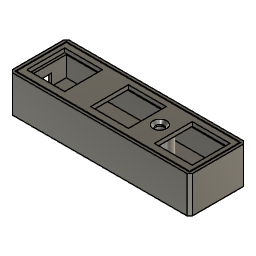
cad (Autodesk Fusion 360 design; units mm, degrees)
Autodesk Fusion 360 part; units mm, degrees
sketch "Sketch1" plane through (0, 0, 0) normal (0, 0, 1) x (1, 0, 0)
  line L0 (0, 0) -> (13.9, 0)
  line L1 (13.9, 0) -> (13.9, 13.9)
  line L2 (13.9, 13.9) -> (0, 13.9)
  line L3 (0, 13.9) -> (0, 0)
  line L4 (0, 6.95) -> (38, 6.95)
  circle A0 centre (42, 6.95) radius 4
  circle A1 centre (42, 6.95) radius 2.5
  line L5 (37.4, 13.9) -> (23.5, 13.9)
  line L6 (37.4, 0) -> (37.4, 13.9)
  line L7 (23.5, 13.9) -> (23.5, 0)
  line L8 (23.5, 0) -> (37.4, 0)
  line L9 (60.9, 13.9) -> (47, 13.9)
  line L10 (60.9, 0) -> (60.9, 13.9)
  line L11 (47, 13.9) -> (47, 0)
  line L12 (47, 0) -> (60.9, 0)
  line L13 (0, 0) -> (0, -0.3232)
  line L14 (0, -0.3232) -> (0, -2.4232)
  line L15 (0, -2.4232) -> (-1.5, -2.4232)
  line L16 (60.9, 13.9) -> (60.9, 16)
  line L17 (60.9, 16) -> (62.4, 16)
  line L18 (62.4, 16) -> (-1.5, 16)
  line L19 (-1.5, 16) -> (-1.5, -2.4232)
  line L20 (-1.5, -2.4232) -> (62.4, -2.4232)
  line L21 (62.4, -2.4232) -> (62.4, 16)
  line L22 (-1.7, -2.6232) -> (62.6, -2.6232)
  line L23 (62.6, -2.6232) -> (62.6, 16.2)
  line L24 (62.6, 16.2) -> (-1.7, 16.2)
  line L25 (-1.7, 16.2) -> (-1.7, -2.6232)
  line L26 (63.6, 17.2) -> (-2.7, 17.2)
  line L27 (-2.7, 17.2) -> (-2.7, -3.6232)
  line L28 (-2.7, -3.6232) -> (63.6, -3.6232)
  line L29 (63.6, -3.6232) -> (63.6, 17.2)
  line L30 (-1.7, -2.6232) -> (-1.7, 5.5768)
  line L31 (-1.7, 5.5768) -> (-1.7, 13.3768)
  circle A2 centre (42, 6.95) radius 1.5
  line L32 (-2.7, 6.7884) -> (-2.7, 2.7884)
  line L33 (-2.7, 2.7884) -> (-1.7, 2.7884)
  line L34 (-1.7, 2.7884) -> (-1.7, 10.7884)
  line L35 (-1.7, 10.7884) -> (-2.7, 10.7884)
  line L36 (-2.7, 10.7884) -> (-2.7, 2.7884)
  line L37 (32.5, 6.7884) -> (32.5, 16.2)
  line L38 (32.5, 16.2) -> (34.5, 16.2)
  line L39 (34.5, 16.2) -> (34.5, -2.3232)
  line L40 (34.5, -2.3232) -> (32.5, -2.3232)
  line L41 (32.5, -2.3232) -> (32.5, 16.2)
  dimension "d1" = 13.9
  dimension "d2" = 13.9
  dimension "d3" = 38
  dimension "d4" = 8
  dimension "d5" = 5
  dimension "d8" = 23.5
  dimension "d9" = 0
  dimension "d10" = 2.1
  dimension "d11" = 1.5
  dimension "d12" = 2.1
  dimension "d13" = 1.5
  dimension "d14" = 0.2
  dimension "d15" = 1.2
  dimension "d18" = 3
  dimension "d47" = 4
  dimension "d48" = 8
  dimension "d58" = 2
  constraint horizontal L0
  constraint vertical L1
  constraint horizontal L2
  constraint vertical L3
  constraint coincident L0.start L3.end
  constraint midpoint L3 L4.start
  constraint perpendicular L1 L4
  constraint coincident L4.end A0
  constraint concentric A0 A1
  constraint perpendicular L0 L13
  constraint perpendicular L0 L14
  constraint perpendicular L14 L15
  constraint perpendicular L9 L16
  constraint perpendicular L16 L17
  constraint horizontal L18
  constraint vertical L19
  constraint horizontal L20
  constraint vertical L21
  constraint perpendicular L22 L30
  constraint parallel L25 L31
  constraint concentric A0 A2
  constraint midpoint L27 L32.start
  constraint perpendicular L28 L32
  constraint horizontal L33
  constraint vertical L34
  constraint horizontal L35
  constraint vertical L36
  constraint coincident L24 L37.end
  constraint perpendicular L18 L37
  constraint horizontal L38
  constraint vertical L39
  constraint horizontal L40
  constraint vertical L41
  measures "d1" distance of L0.start L0.end
  measures "d2" distance of L0.start L2.end
  measures "d3" distance of L4.start L4.end
  measures "d4" diameter of A0
  measures "d5" diameter of A1
  measures "d10" distance of L13.end L14.end
  measures "d11" distance of L14.end L15.end
  measures "d12" distance of L9.start L16.end
  measures "d13" distance of L16.end L17.end
  measures "d18" diameter of A2
  measures "d47" distance of L32.start L32.end
  measures "d48" distance of L32.end L35.end
  measures "d58" distance of L37.end L38.end
extrude "Extrude1" add sketch "Sketch1" along normal blind 1.5 contours L1 L2 L3 L4 L5 L7 L13 L14 L15 L18 L19 L20 L37 L41 | L0 L1 L4 L5 L6 L7 L8 L13 L14 L17 L18 L20 L21 L39 L40 L41 | L5 L18 L37 L39 L41 | L8 L39 L40 L41 | A0 | A1 makes body 1
extrude "Extrude2" add sketch "Sketch1" along normal blind 1.5 and the other way blind 20 separate body contours L22 L23 L24 L25 L26 L27 L28 L29 L30 L31 L33 L35 L38 | L25 L27 L30 L31 L32 L33 L34 L35 L36 makes body 2
extrude "Extrude3" add sketch "Sketch1" along normal blind -22 and the other way blind 20 contours L0 L1 L3 L4 | L1 L2 L3 L4 L5 L7 L13 L14 L15 L18 L19 L20 L37 L41 | L0 L1 L4 L5 L6 L7 L8 L13 L14 L17 L18 L20 L21 L39 L40 L41 | L1 L2 L3 L4 | L15 L17 L18 L19 L20 L21 L22 L23 L24 L25 L30 L31 L34 L37 L39 L41 | L4 L5 L7 L37 L41 | L4 L7 L8 L37 L41 | L4 L5 L37 L39 L41 | L4 L8 L37 L39 L41 | L4 L5 L6 L39 | L4 L6 L8 L39 | L5 L18 L37 L39 L41 | L8 L39 L40 L41 | L18 L24 L37 L38 L39 L41 | L22 L23 L24 L25 L26 L27 L28 L29 L30 L31 L33 L35 L38 | L25 L27 L30 L31 L32 L33 L34 L35 L36 | A0 | A1 | L9 L10 L11 L12 | A2 bodies 2
extrude "Extrude4" cut sketch "Sketch1" along normal blind -11 and the other way blind 7 contours L0 L1 L3 L4 | L1 L2 L3 L4 L5 L7 L13 L14 L15 L18 L19 L20 L37 L41 | L0 L1 L4 L5 L6 L7 L8 L13 L14 L17 L18 L20 L21 L39 L40 L41 | L1 L2 L3 L4 | L15 L17 L18 L19 L20 L21 L22 L23 L24 L25 L30 L31 L34 L37 L39 L41 | L4 L5 L7 L37 L41 | L4 L7 L8 L37 L41 | L4 L5 L37 L39 L41 | L4 L8 L37 L39 L41 | L4 L5 L6 L39 | L4 L6 L8 L39 | L5 L18 L37 L39 L41 | L8 L39 L40 L41 | L18 L24 L37 L38 L39 L41 | A0 | A1 | L9 L10 L11 L12 | A2 bodies 2
extrude "Extrude5" add sketch "Sketch1" along normal blind -20 and the other way blind 0.5 contours A0 bodies 2
extrude "Extrude6" add sketch "Sketch1" along normal blind -2 and the other way blind 0.2 contours L15 L17 L18 L19 L20 L21 L22 L23 L24 L25 L30 L31 L34 L37 L39 L41 | L18 L24 L37 L38 L39 L41 bodies 2
extrude "Extrude7" add 1 faces at (19.8, -2.4232, -1.4) along direction (0, 1, 0) blind 0.4 on bodies 2 bodies 2
extrude "Extrude8" add 1 faces at (19.8, 16, -0.8) along direction (0, -1, 0) blind 0.4 on bodies 2 bodies 2
chamfer "Chamfer1" distance 1 angle 45 4 edges at (-2.7, 17.2, -10.25) (-2.7, -3.6232, -10.25) (63.6, -3.6232, -10.25) (63.6, 17.2, -10.25) on bodies 2
chamfer "Chamfer2" distance 1 angle 45 1 edges at (40.6015, 7.4924, 1.5) on bodies 1
extrude "Extrude9" add 1 faces at (11.5333, 6.8423, -20) along direction (0, 0, 1) blind 10 on bodies 2 bodies 2
extrude "Extrude10" cut 1 faces at (19.7333, 10.2589, -22) along direction (0, 0, 1) blind 10 on bodies 2 bodies 2
extrude "Extrude11" cut sketch "Sketch1" along normal blind -9 and the other way blind 6 contours L25 L27 L30 L31 L32 L33 L34 L35 L36 bodies 2
extrude "Extrude12" add sketch "Sketch1" along normal blind -10 and the other way blind 7.5 contours L0 L1 L4 L5 L6 L7 L8 L13 L14 L17 L18 L20 L21 L39 L40 L41 | L4 L5 L37 L39 L41 | L4 L8 L37 L39 L41 | L5 L18 L37 L39 L41 | L8 L39 L40 L41 | L18 L24 L37 L38 L39 L41 bodies 2
extrude "Extrude13" add sketch "Sketch1" along normal blind -12 and the other way blind 8 contours A1 | A2 bodies 2
extrude "Extrude14" cut 1 faces at (41.6333, 7.0053, -8) along direction (0, 0, -1) blind 2 on bodies 2 bodies 2
extrude "Extrude15" cut sketch "Sketch1" along normal blind -10 and the other way blind 7.5 contours L0 L1 L4 L5 L6 L7 L8 L13 L14 L17 L18 L20 L21 L39 L40 L41 | L9 L10 L11 L12 bodies 2
extrude "Extrude16" add 1 faces at (62.4, 9.7256, -0.8) along direction (-1, 0, 0) blind 0.4 on bodies 2 bodies 2
extrude "Extrude17" add 1 faces at (-1.5, 9.7256, -1.4) along direction (1, 0, 0) blind 0.4 on bodies 2 bodies 2
extrude "Extrude18" cut 1 faces at (-2.3667, 8.1217, -9) along direction (0, 0, -1) blind 0.2 on bodies 2 bodies 2
extrude "Extrude19" cut 1 faces at (-2.3667, 8.1217, -6) along direction (0, 0, 1) blind 0.2 on bodies 2 bodies 2
named bodies: "top", "bottom"
